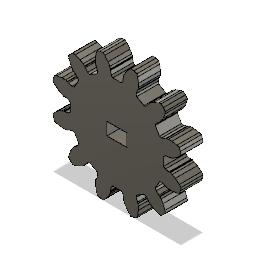
Motor Gear (Autodesk Fusion 360 design; units mm, degrees)
Autodesk Fusion 360 part; units mm, degrees
(part 1 of 2)
sketch "Sketch1" plane through (0, 0, 0) normal (0, 0, 1) x (1, 0, 0)
  circle A0 centre (141.6354, 183.0412) radius 17.7716
  line L0 (144.3354, 181.3412) -> (138.9354, 181.3412)
  line L1 (138.9354, 181.3412) -> (138.9354, 184.7412)
  line L2 (138.9354, 184.7412) -> (144.3354, 184.7412)
  line L3 (144.3354, 184.7412) -> (144.3354, 181.3412)
  line L4 (144.3354, 181.3412) -> (138.9354, 184.7412) construction
  line L5 (138.9354, 181.3412) -> (144.3354, 184.7412) construction
  line L6 (110, 165) -> (115.5, 165)
  line L7 (115.5, 165) -> (115.5, 168.5)
  line L8 (115.5, 168.5) -> (110, 168.5)
  line L9 (110, 168.5) -> (110, 165)
  line L10 (107, 171) -> (118, 171)
  line L11 (118, 171) -> (118, 162)
  line L12 (118, 162) -> (107, 162)
  line L13 (107, 162) -> (107, 171)
  arc A1 (143.6355, 181.3412) -> (143.8567, 181.6426) centre (141.6354, 183.0412) ccw
  arc A2 (143.8567, 184.4399) -> (143.6355, 184.7412) centre (141.6354, 183.0412) ccw
  arc A3 (139.6352, 184.7412) -> (139.414, 184.4399) centre (141.6354, 183.0412) ccw
  arc A4 (139.414, 181.6426) -> (139.6352, 181.3412) centre (141.6354, 183.0412) ccw
  point P0 (145.415, 200.4062)
  point P1 (137.8557, 165.6762)
  point P2 (141.6354, 183.0412)
  dimension "d1" = 5.25
  dimension "d6" = 5.4
  dimension "d7" = 3.4
  dimension "d8" = 5.5
  dimension "d9" = 3.5
  constraint coincident A0 P1
  constraint coincident A0 P0
  constraint concentric A0 A1
  constraint perpendicular L0 L1
  constraint parallel L0 L2
  constraint parallel L1 L3
  constraint horizontal L0
  constraint coincident L4 P2
  constraint coincident L5 P2
  constraint coincident P2 A0.centre
  constraint horizontal L6
  constraint vertical L7
  constraint horizontal L8
  constraint vertical L9
  constraint horizontal L10
  constraint vertical L11
  constraint horizontal L12
  constraint vertical L13
  constraint coincident L0 A4.end
  constraint coincident L0 A1.start
  constraint coincident L2 A2.end
  constraint coincident L2 A3.start
  constraint concentric A1 A3
  constraint coincident L4 A1.end
  constraint coincident L5 A2.start
  constraint concentric A1 A2
  constraint coincident L4 A3.end
  constraint coincident L5 A4.start
  constraint concentric A3 A4
  measures "d1" diameter of A1
  measures "d6" distance of L1.end L2.end
  measures "d7" distance of L0.end L1.end
  measures "d8" distance of L6.start L6.end
  measures "d9" distance of L6.start L8.end
sketch "30_12_Gears" plane through (0, 0, 0) normal (0, 0, 1) x (1, 0, 0)
  line L0 (152.0494, 175.714) -> (153.1879, 177.6861)
  line L1 (146.2489, 165.8233) -> (147.0446, 166.1129)
  line L2 (154.7859, 181.4961) -> (154.3178, 181.9027)
  line L3 (154.7841, 171.0855) -> (154.6561, 171.7367)
  line L4 (153.297, 174.2848) -> (153.2284, 174.3402)
  line L5 (154.2398, 170.4368) -> (154.7841, 171.0855)
  line L6 (150.2112, 171.6754) -> (150.3365, 171.4483)
  line L7 (142.7739, 170.3589) -> (143.1805, 169.8908)
  line L8 (154.9672, 177.352) -> (155.0495, 177.3202)
  line L9 (146.8725, 170.88) -> (146.9906, 171.4887)
  line L10 (156.5401, 177.1992) -> (157.9358, 177.4173)
  line L11 (156.1128, 181.2888) -> (156.0257, 181.3023)
  line L12 (158.8534, 178.4278) -> (159.0004, 179.2617)
  line L13 (153.0013, 174.4654) -> (152.2515, 175.1279)
  line L14 (152.2515, 175.1279) -> (152.0494, 175.714)
  line L15 (156.0257, 181.3023) -> (155.7665, 181.2973)
  line L16 (147.3246, 169.7094) -> (147.1906, 169.9314)
  line L17 (144.0283, 167.2123) -> (144.9151, 166.1127)
  line L18 (145.415, 165.6762) -> (146.2489, 165.8233)
  line L19 (147.4775, 168.1365) -> (147.4585, 169.1075)
  line L20 (151.6222, 170.5295) -> (152.94, 170.0205)
  line L21 (143.3743, 168.6509) -> (143.3879, 168.5638)
  line L22 (140.0902, 169.8908) -> (140.4968, 170.3589)
  line L23 (140.4968, 170.3589) -> (142.7739, 170.3589)
  line L24 (153.5912, 169.8926) -> (154.2398, 170.4368)
  line L25 (154.1472, 173.0544) -> (153.6453, 173.8858)
  line L26 (158.5637, 177.6321) -> (158.8534, 178.4278)
  line L27 (158.564, 179.7616) -> (157.4643, 180.6484)
  line L28 (154.6561, 171.7367) -> (154.1472, 173.0544)
  line L29 (153.2284, 174.3402) -> (153.0013, 174.4654)
  line L30 (155.0495, 177.3202) -> (155.5692, 177.2181)
  line L31 (147.2594, 166.7408) -> (147.4775, 168.1365)
  line L32 (148.9626, 172.6273) -> (149.5488, 172.4252)
  line L33 (147.3564, 169.6272) -> (147.3246, 169.7094)
  line L34 (147.4585, 169.1075) -> (147.3564, 169.6272)
  line L35 (156.614, 181.1174) -> (156.1128, 181.2888)
  line L36 (143.3793, 168.9102) -> (143.3743, 168.6509)
  line L37 (153.7966, 177.8041) -> (154.7452, 177.486)
  line L38 (143.1805, 169.8908) -> (143.3793, 168.9102)
  line L39 (144.9151, 166.1127) -> (145.415, 165.6762)
  line L40 (154.7452, 177.486) -> (154.9672, 177.352)
  line L41 (159.0004, 179.2617) -> (158.564, 179.7616)
  line L42 (155.5692, 177.2181) -> (156.5401, 177.1992)
  line L43 (153.6453, 173.8858) -> (153.297, 174.2848)
  line L44 (149.5488, 172.4252) -> (150.2112, 171.6754)
  line L45 (143.5593, 168.0627) -> (144.0283, 167.2123)
  line L46 (153.1879, 177.6861) -> (153.7966, 177.8041)
  line L47 (155.7665, 181.2973) -> (154.7859, 181.4961)
  line L48 (154.3178, 181.9027) -> (154.3178, 184.1798)
  line L49 (157.9358, 177.4173) -> (158.5637, 177.6321)
  line L50 (154.3178, 184.1798) -> (154.7859, 184.5864)
  line L51 (154.7859, 184.5864) -> (155.7665, 184.7852)
  line L52 (155.7665, 184.7852) -> (156.0257, 184.7801)
  line L53 (156.0257, 184.7801) -> (156.1128, 184.7937)
  line L54 (156.1128, 184.7937) -> (156.614, 184.9651)
  line L55 (140.4968, 195.7236) -> (140.0902, 196.1917)
  line L56 (145.415, 200.4062) -> (144.9151, 199.9698)
  line L57 (144.0283, 198.8702) -> (143.5593, 198.0198)
  line L58 (139.8829, 197.5187) -> (139.7115, 198.0198)
  line L59 (147.3246, 196.3731) -> (147.3564, 196.4553)
  line L60 (139.8914, 197.1723) -> (139.8965, 197.4316)
  line L61 (155.0495, 188.7622) -> (154.9672, 188.7305)
  line L62 (151.6222, 195.553) -> (150.7908, 195.0511)
  line L63 (152.2515, 190.9546) -> (153.0013, 191.6171)
  line L64 (150.3365, 194.6342) -> (150.2112, 194.4071)
  line L65 (154.9672, 188.7305) -> (154.7452, 188.5965)
  line L66 (153.0013, 191.6171) -> (153.2284, 191.7423)
  line L67 (157.4643, 180.6484) -> (156.614, 181.1174)
  line L68 (150.3918, 194.7028) -> (150.3365, 194.6342)
  line L69 (153.6453, 192.1967) -> (154.1472, 193.0281)
  line L70 (159.0004, 186.8208) -> (158.8534, 187.6547)
  line L71 (150.7908, 195.0511) -> (150.3918, 194.7028)
  line L72 (153.7966, 188.2783) -> (153.1879, 188.3964)
  line L73 (154.2398, 195.6457) -> (153.5912, 196.1899)
  line L74 (152.94, 196.062) -> (151.6222, 195.553)
  line L75 (147.1906, 196.1511) -> (147.3246, 196.3731)
  line L76 (148.9626, 193.4552) -> (146.9906, 194.5938)
  line L77 (153.2284, 191.7423) -> (153.297, 191.7977)
  line L78 (153.297, 191.7977) -> (153.6453, 192.1967)
  line L79 (153.5912, 196.1899) -> (152.94, 196.062)
  line L80 (143.5593, 198.0198) -> (143.3879, 197.5187)
  line L81 (158.5637, 188.4504) -> (157.9358, 188.6652)
  line L82 (155.5692, 188.8644) -> (155.0495, 188.7622)
  line L83 (156.614, 184.9651) -> (157.4643, 185.4341)
  line L84 (149.5488, 193.6573) -> (148.9626, 193.4552)
  line L85 (146.9906, 194.5938) -> (146.8725, 195.2025)
  line L86 (156.5401, 188.8833) -> (155.5692, 188.8644)
  line L87 (154.7452, 188.5965) -> (153.7966, 188.2783)
  line L88 (140.0902, 196.1917) -> (139.8914, 197.1723)
  line L89 (158.8534, 187.6547) -> (158.5637, 188.4504)
  line L90 (154.1472, 193.0281) -> (154.6561, 194.3458)
  line L91 (154.6561, 194.3458) -> (154.7841, 194.997)
  line L92 (150.2112, 194.4071) -> (149.5488, 193.6573)
  line L93 (152.0494, 190.3685) -> (152.2515, 190.9546)
  line L94 (154.7841, 194.997) -> (154.2398, 195.6457)
  line L95 (157.9358, 188.6652) -> (156.5401, 188.8833)
  line L96 (153.1879, 188.3964) -> (152.0494, 190.3685)
  line L97 (157.4643, 185.4341) -> (158.564, 186.3209)
  line L98 (158.564, 186.3209) -> (159.0004, 186.8208)
  line L99 (146.8725, 195.2025) -> (147.1906, 196.1511)
  line L100 (147.3564, 196.4553) -> (147.4585, 196.975)
  line L101 (142.7739, 195.7236) -> (140.4968, 195.7236)
  line L102 (147.4775, 197.946) -> (147.2594, 199.3417)
  line L103 (129.9738, 191.7977) -> (130.0424, 191.7423)
  line L104 (130.3307, 196.062) -> (129.6796, 196.1899)
  line L105 (133.0595, 194.4071) -> (132.9342, 194.6342)
  line L106 (133.722, 193.6573) -> (133.0595, 194.4071)
  line L107 (124.707, 188.4504) -> (124.707, 188.4504)
  line L108 (130.2695, 191.6171) -> (131.0193, 190.9546)
  line L109 (127.7016, 188.8644) -> (126.7306, 188.8833)
  line L110 (124.707, 188.4504) -> (124.707, 188.4504)
  line L111 (131.0193, 190.9546) -> (131.2214, 190.3685)
  line L112 (136.2802, 194.5938) -> (134.3081, 193.4552)
  line L113 (128.4866, 194.997) -> (128.6146, 194.3458)
  line L114 (131.2214, 190.3685) -> (130.0828, 188.3964)
  line L115 (131.6485, 195.553) -> (130.3307, 196.062)
  line L116 (143.3743, 197.4316) -> (143.3793, 197.1723)
  line L117 (134.3081, 193.4552) -> (133.722, 193.6573)
  line L118 (139.7115, 198.0198) -> (139.2424, 198.8702)
  line L119 (144.9151, 199.9698) -> (144.0283, 198.8702)
  line L120 (146.2489, 200.2592) -> (145.415, 200.4062)
  line L121 (132.9342, 194.6342) -> (132.8789, 194.7028)
  line L122 (136.0114, 199.3417) -> (135.7933, 197.946)
  line L123 (139.8965, 197.4316) -> (139.8829, 197.5187)
  line L124 (132.8789, 194.7028) -> (132.4799, 195.0511)
  line L125 (129.4741, 188.2783) -> (128.5255, 188.5965)
  line L126 (130.0828, 188.3964) -> (129.4741, 188.2783)
  line L127 (147.4585, 196.975) -> (147.4775, 197.946)
  line L128 (128.6146, 194.3458) -> (129.1236, 193.0281)
  line L129 (130.0424, 191.7423) -> (130.2695, 191.6171)
  line L130 (138.3557, 199.9698) -> (137.8557, 200.4062)
  line L131 (135.9461, 196.3731) -> (136.0801, 196.1511)
  line L132 (139.2424, 198.8702) -> (138.3557, 199.9698)
  line L133 (143.3793, 197.1723) -> (143.1805, 196.1917)
  line L134 (137.8557, 200.4062) -> (137.0218, 200.2592)
  line L135 (143.3879, 197.5187) -> (143.3743, 197.4316)
  line L136 (136.2261, 199.9696) -> (136.0114, 199.3417)
  line L137 (135.7933, 197.946) -> (135.8122, 196.975)
  line L138 (129.6796, 196.1899) -> (129.0309, 195.6457)
  line L139 (147.0446, 199.9696) -> (146.2489, 200.2592)
  line L140 (143.1805, 196.1917) -> (142.7739, 195.7236)
  line L141 (147.2594, 199.3417) -> (147.0446, 199.9696)
  line L142 (137.0218, 200.2592) -> (136.2261, 199.9696)
  line L143 (129.1236, 193.0281) -> (129.6255, 192.1967)
  line L144 (128.5255, 188.5965) -> (128.3035, 188.7305)
  line L145 (135.8122, 196.975) -> (135.9143, 196.4553)
  line L146 (136.0801, 196.1511) -> (136.3982, 195.2025)
  line L147 (129.0309, 195.6457) -> (128.4866, 194.997)
  line L148 (132.4799, 195.0511) -> (131.6485, 195.553)
  line L149 (128.3035, 188.7305) -> (128.2213, 188.7622)
  line L150 (135.9143, 196.4553) -> (135.9461, 196.3731)
  line L151 (129.6255, 192.1967) -> (129.9738, 191.7977)
  line L152 (136.3982, 195.2025) -> (136.2802, 194.5938)
  line L153 (128.2213, 188.7622) -> (127.7016, 188.8644)
  line L154 (126.7306, 188.8833) -> (125.3349, 188.6652)
  line L155 (124.5194, 177.6472) -> (123.9642, 177.8157)
  line L156 (123.8799, 180.6066) -> (124.2682, 180.7082)
  line L157 (125.0362, 177.45) -> (124.5194, 177.6472)
  line L158 (126.4909, 176.7057) -> (125.6979, 177.1431)
  line L159 (123.6055, 177.9958) -> (123.446, 178.1876)
  line L160 (124.2682, 180.7082) -> (124.8463, 180.7576)
  line L161 (125.6979, 177.1431) -> (125.0362, 177.45)
  line L162 (125.3928, 180.843) -> (126.1039, 181.0056)
  line L163 (127.7577, 173.6189) -> (128.0126, 174.5701)
  line L164 (128.0126, 174.5701) -> (128.1667, 175.5427)
  line L165 (127.3994, 176.1183) -> (126.4909, 176.7057)
  line L166 (125.3349, 188.6652) -> (124.707, 188.4504)
  line L167 (124.8463, 180.7576) -> (125.3928, 180.843)
  line L168 (123.9642, 177.8157) -> (123.6055, 177.9958)
  line L169 (128.1667, 175.5427) -> (127.3994, 176.1183)
  line L170 (123.446, 178.1876) -> (123.684, 180.4522)
  line L171 (123.684, 180.4522) -> (123.8799, 180.6066)
  line L172 (123.5698, 192.9026) -> (122.9941, 192.8307)
  line L173 (125.0362, 188.6323) -> (125.6979, 188.9392)
  line L174 (128.8514, 182.0578) -> (128.903, 183.0412)
  line L175 (122.5932, 192.8493) -> (122.3694, 192.9596)
  line L176 (124.2682, 185.3741) -> (123.8799, 185.4758)
  line L177 (128.1667, 190.5397) -> (128.0126, 191.5122)
  line L178 (127.9813, 181.6542) -> (128.8514, 182.0578)
  line L179 (127.9813, 184.4281) -> (126.9705, 184.8137)
  line L180 (123.8799, 185.4758) -> (123.684, 185.6301)
  line L181 (126.9705, 181.2686) -> (127.9813, 181.6542)
  line L182 (126.1039, 181.0056) -> (126.9705, 181.2686)
  line L183 (125.7538, 192.8443) -> (124.8515, 192.9214)
  line L184 (128.903, 183.0412) -> (128.8514, 184.0246)
  line L185 (126.9705, 184.8137) -> (126.1039, 185.0767)
  line L186 (126.1039, 185.0767) -> (125.3928, 185.2393)
  line L187 (124.5194, 188.4352) -> (125.0362, 188.6323)
  line L188 (123.446, 187.8948) -> (123.6055, 188.0865)
  line L189 (124.8515, 192.9214) -> (124.1222, 192.9327)
  line L190 (125.6979, 188.9392) -> (126.4909, 189.3766)
  line L191 (123.9642, 188.2667) -> (124.5194, 188.4352)
  line L192 (126.4909, 189.3766) -> (127.3994, 189.964)
  line L193 (124.1222, 192.9327) -> (123.5698, 192.9026)
  line L194 (126.8227, 192.6773) -> (125.7538, 192.8443)
  line L195 (125.3928, 185.2393) -> (124.8463, 185.3247)
  line L196 (122.9941, 192.8307) -> (122.5932, 192.8493)
  line L197 (124.8463, 185.3247) -> (124.2682, 185.3741)
  line L198 (123.6055, 188.0865) -> (123.9642, 188.2667)
  line L199 (128.0126, 191.5122) -> (127.7577, 192.4634)
  line L200 (122.3694, 192.9596) -> (121.6657, 195.1252)
  line L201 (114.0546, 208.3143) -> (114.4047, 208.7769)
  line L202 (115.4463, 210.6974) -> (115.8361, 211.7066)
  line L203 (116.4975, 206.4527) -> (116.0007, 206.1528)
  line L204 (112.0365, 212.6016) -> (111.4399, 212.182)
  line L205 (110.2518, 211.2158) -> (110.006, 211.1735)
  line L206 (110.006, 211.1735) -> (108.1637, 212.512)
  line L207 (110.5871, 211.4364) -> (110.2518, 211.2158)
  line L208 (115.3776, 206.0166) -> (113.8539, 207.7088)
  line L209 (119.182, 202.7578) -> (119.5739, 203.1482)
  line L210 (118.4889, 202.0676) -> (118.7433, 202.3781)
  line L211 (113.8703, 207.9577) -> (114.0546, 208.3143)
  line L212 (124.9334, 200.4905) -> (123.9744, 200.5053)
  line L213 (113.8539, 207.7088) -> (113.8703, 207.9577)
  line L214 (108.128, 212.7588) -> (108.2341, 213.1459)
  line L215 (116.0007, 206.1528) -> (115.6269, 206.0068)
  line L216 (118.7433, 202.3781) -> (119.182, 202.7578)
  line L217 (120.6001, 204.4198) -> (121.1912, 205.3259)
  line L218 (122.0953, 195.5967) -> (122.6034, 195.877)
  line L219 (123.9744, 200.5053) -> (122.8941, 200.4464)
  line L220 (121.1912, 205.3259) -> (121.6579, 206.1638)
  line L221 (120.1975, 199.8592) -> (119.8015, 199.7942)
  line L222 (121.1216, 206.9897) -> (120.5019, 207.755)
  line L223 (119.5597, 199.8555) -> (118.4211, 201.8275)
  line L224 (111.0107, 211.8329) -> (110.5871, 211.4364)
  line L225 (120.0536, 203.6977) -> (120.6001, 204.4198)
  line L226 (122.8941, 200.4464) -> (121.9955, 200.3342)
  line L227 (118.5163, 207.2878) -> (117.6607, 206.9912)
  line L228 (121.7819, 195.346) -> (122.0953, 195.5967)
  line L229 (123.0679, 196.1773) -> (123.6513, 196.6151)
  line L230 (118.4211, 201.8275) -> (118.4889, 202.0676)
  line L231 (121.9955, 200.3342) -> (121.2798, 200.1935)
  line L232 (121.2798, 200.1935) -> (120.7457, 200.0493)
  line L233 (123.684, 185.6301) -> (123.446, 187.8948)
  line L234 (124.336, 197.2078) -> (125.1026, 197.9712)
  line L235 (125.3805, 199.6131) -> (124.9334, 200.4905)
  line L236 (121.6657, 195.1252) -> (121.7819, 195.346)
  line L237 (125.1026, 197.9712) -> (125.7334, 198.6938)
  line L238 (119.5739, 203.1482) -> (120.0536, 203.6977)
  line L239 (120.7457, 200.0493) -> (120.1975, 199.8592)
  line L240 (121.6579, 206.1638) -> (121.1216, 206.9897)
  line L241 (120.5019, 207.755) -> (119.5607, 207.57)
  line L242 (119.8015, 199.7942) -> (119.5597, 199.8555)
  line L243 (125.7334, 198.6938) -> (125.3805, 199.6131)
  line L244 (127.3994, 189.964) -> (128.1667, 190.5397)
  line L245 (115.0619, 209.8775) -> (115.4463, 210.6974)
  line L246 (127.7577, 192.4634) -> (126.8227, 192.6773)
  line L247 (128.8514, 184.0246) -> (127.9813, 184.4281)
  line L248 (122.6034, 195.877) -> (123.0679, 196.1773)
  line L249 (119.5607, 207.57) -> (118.5163, 207.2878)
  line L250 (123.6513, 196.6151) -> (124.336, 197.2078)
  line L251 (94.15, 220.5651) -> (93.979, 221.4545)
  line L252 (96.8821, 217.7658) -> (96.6748, 217.6272)
  line L253 (101.5993, 216.0271) -> (101.513, 216.2612)
  line L254 (108.8944, 214.8844) -> (109.1, 215.7664)
  line L255 (85.8653, 221.825) -> (85.3761, 222.79)
  line L256 (94.2374, 219.841) -> (94.15, 220.5651)
  line L257 (93.979, 221.4545) -> (93.7012, 222.5)
  line L258 (115.4221, 213.3196) -> (114.6568, 213.9393)
  line L259 (99.7986, 222.0456) -> (99.1459, 221.3427)
  line L260 (108.5311, 218.3262) -> (107.6537, 218.7733)
  line L261 (101.513, 216.2612) -> (101.5363, 216.6619)
  line L262 (82.3396, 221.4545) -> (82.1686, 220.5651)
  line L263 (104.1934, 215.4789) -> (103.9112, 215.1934)
  line L264 (109.357, 217.7899) -> (108.5311, 218.3262)
  line L265 (111.4399, 212.182) -> (111.0107, 211.8329)
  line L266 (113.7747, 213.5627) -> (112.8118, 213.0696)
  line L267 (104.8724, 216.3855) -> (104.5252, 215.9548)
  line L268 (93.7012, 222.5) -> (93.3908, 223.4076)
  line L269 (107.6537, 218.7733) -> (106.8692, 218.2215)
  line L270 (108.6797, 214.1873) -> (108.8944, 214.8844)
  line L271 (112.8118, 213.0696) -> (112.0365, 212.6016)
  line L272 (109.2714, 216.8345) -> (109.357, 217.7899)
  line L273 (105.3688, 216.9199) -> (104.8724, 216.3855)
  line L274 (101.6691, 221.4378) -> (100.7498, 221.7907)
  line L275 (101.8384, 219.4051) -> (101.784, 220.4855)
  line L276 (101.5363, 216.6619) -> (101.668, 217.2269)
  line L277 (116.9898, 206.7049) -> (116.4975, 206.4527)
  line L278 (96.6748, 217.6272) -> (94.4474, 218.1006)
  line L279 (115.8361, 211.7066) -> (116.1184, 212.6233)
  line L280 (106.8692, 218.2215) -> (106.0298, 217.5389)
  line L281 (101.784, 220.4855) -> (101.6691, 221.4378)
  line L282 (94.4474, 218.1006) -> (94.3144, 218.3116)
  line L283 (114.6569, 213.9393) -> (113.7747, 213.5627)
  line L284 (108.4804, 213.6713) -> (108.6797, 214.1873)
  line L285 (97.0988, 218.1037) -> (96.8821, 217.7658)
  line L286 (101.7557, 217.7731) -> (101.8207, 218.4996)
  line L287 (89.7231, 219.7659) -> (89.6135, 219.1961)
  line L288 (98.4668, 220.5006) -> (97.9489, 219.7577)
  line L289 (90.4533, 221.825) -> (90.1012, 220.9907)
  line L290 (106.0298, 217.5389) -> (105.3688, 216.9199)
  line L291 (90.1012, 220.9907) -> (89.8651, 220.3005)
  line L292 (94.2539, 218.7084) -> (94.2652, 219.2885)
  line L293 (90.9425, 222.79) -> (90.4533, 221.825)
  line L294 (101.668, 217.2269) -> (101.7557, 217.7731)
  line L295 (117.6607, 206.9912) -> (116.9898, 206.7049)
  line L296 (97.9489, 219.7577) -> (97.5745, 219.1317)
  line L297 (97.3244, 218.6383) -> (97.0988, 218.1037)
  line L298 (104.5252, 215.9548) -> (104.1934, 215.4789)
  line L299 (92.4182, 223.5616) -> (91.4348, 223.6132)
  line L300 (103.6795, 215.1009) -> (101.5993, 216.0271)
  line L301 (87.0207, 218.6419) -> (86.8467, 218.8206)
  line L302 (108.2341, 213.1459) -> (108.4804, 213.6713)
  line L303 (116.1184, 212.6233) -> (115.4221, 213.3196)
  line L304 (108.1637, 212.512) -> (108.128, 212.7588)
  line L305 (115.6269, 206.0068) -> (115.3776, 206.0166)
  line L306 (99.1459, 221.3427) -> (98.4668, 220.5006)
  line L307 (101.8207, 218.4996) -> (101.8384, 219.4051)
  line L308 (114.707, 209.2402) -> (115.0619, 209.8775)
  line L309 (114.4047, 208.7769) -> (114.707, 209.2402)
  line L310 (109.1, 215.7664) -> (109.2714, 216.8345)
  line L311 (97.5745, 219.1317) -> (97.3244, 218.6383)
  line L312 (100.7498, 221.7907) -> (99.7986, 222.0456)
  line L313 (103.9112, 215.1934) -> (103.6795, 215.1009)
  line L314 (85.3761, 222.79) -> (84.8838, 223.6132)
  line L315 (74.5629, 148.3094) -> (74.4978, 147.5829)
  line L316 (94.4474, 147.9819) -> (96.6748, 148.4554)
  line L317 (82.0647, 147.3741) -> (82.0534, 146.794)
  line L318 (93.3908, 142.675) -> (93.7012, 143.5825)
  line L319 (75.5688, 144.2918) -> (76.52, 144.037)
  line L320 (86.2174, 145.0919) -> (86.4534, 145.782)
  line L321 (82.0534, 146.794) -> (82.0812, 146.2415)
  line L322 (82.9278, 142.675) -> (83.9004, 142.5209)
  line L323 (82.3396, 144.6281) -> (82.6174, 143.5825)
  line L324 (78.7441, 146.9509) -> (78.9942, 147.4443)
  line L325 (81.8712, 147.9819) -> (82.0042, 147.7709)
  line L326 (74.6495, 144.6447) -> (75.5688, 144.2918)
  line L327 (78.9942, 147.4443) -> (79.2198, 147.9788)
  line L328 (74.5346, 145.597) -> (74.6495, 144.6447)
  line L329 (74.4802, 146.6775) -> (74.5346, 145.597)
  line L330 (74.6506, 148.8556) -> (74.5629, 148.3094)
  line L331 (82.6174, 143.5825) -> (82.9278, 142.675)
  line L332 (82.0042, 147.7709) -> (82.0647, 147.3741)
  line L333 (85.8653, 144.2575) -> (86.2174, 145.0919)
  line L334 (83.9004, 142.5209) -> (84.8838, 142.4694)
  line L335 (85.3761, 143.2926) -> (85.8653, 144.2575)
  line L336 (76.52, 144.037) -> (77.1727, 144.7398)
  line L337 (78.3697, 146.3249) -> (78.7441, 146.9509)
  line L338 (74.4978, 147.5829) -> (74.4802, 146.6775)
  line L339 (77.1727, 144.7398) -> (77.8518, 145.582)
  line L340 (86.4534, 145.782) -> (86.5955, 146.3166)
  line L341 (86.5955, 146.3166) -> (86.705, 146.8864)
  line L342 (91.4348, 142.4694) -> (92.4182, 142.5209)
  line L343 (82.1686, 145.5174) -> (82.3396, 144.6281)
  line L344 (82.0812, 146.2415) -> (82.1686, 145.5174)
  line L345 (79.2198, 147.9788) -> (79.4364, 148.3167)
  line L346 (93.979, 144.6281) -> (94.15, 145.5174)
  line L347 (77.8518, 145.582) -> (78.3697, 146.3249)
  line L348 (79.6438, 148.4554) -> (81.8712, 147.9819)
  line L349 (84.8838, 142.4694) -> (85.3761, 143.2926)
  line L350 (79.4364, 148.3167) -> (79.6438, 148.4554)
  line L351 (89.7231, 146.3166) -> (89.8651, 145.782)
  line L352 (86.8467, 147.2619) -> (87.0207, 147.4407)
  line L353 (94.15, 145.5174) -> (94.2374, 146.2415)
  line L354 (103.6795, 150.9816) -> (103.9112, 150.8891)
  line L355 (107.6537, 147.3093) -> (108.5311, 147.7563)
  line L356 (97.5745, 146.9509) -> (97.9489, 146.3249)
  line L357 (108.5311, 147.7563) -> (109.357, 148.2926)
  line L358 (101.6691, 144.6447) -> (101.784, 145.597)
  line L359 (97.0988, 147.9788) -> (97.3244, 147.4443)
  line L360 (86.705, 146.8864) -> (86.8467, 147.2619)
  line L361 (94.2652, 146.794) -> (94.2539, 147.3741)
  line L362 (89.4719, 147.2619) -> (89.6135, 146.8864)
  line L363 (96.6748, 148.4554) -> (96.8821, 148.3167)
  line L364 (97.9489, 146.3249) -> (98.4668, 145.582)
  line L365 (109.2714, 149.248) -> (109.1, 150.3162)
  line L366 (99.7986, 144.037) -> (100.7498, 144.2918)
  line L367 (104.5252, 150.1277) -> (104.8724, 149.6971)
  line L368 (94.2374, 146.2415) -> (94.2652, 146.794)
  line L369 (109.1, 150.3162) -> (108.8944, 151.1982)
  line L370 (101.513, 149.8214) -> (101.5993, 150.0554)
  line L371 (108.4804, 152.4113) -> (108.2341, 152.9366)
  line L372 (104.1934, 150.6037) -> (104.5252, 150.1277)
  line L373 (89.6135, 146.8864) -> (89.7231, 146.3166)
  line L374 (94.3144, 147.7709) -> (94.4474, 147.9819)
  line L375 (97.3244, 147.4443) -> (97.5745, 146.9509)
  line L376 (90.9425, 143.2926) -> (91.4348, 142.4694)
  line L377 (99.1459, 144.7398) -> (99.7986, 144.037)
  line L378 (98.4668, 145.582) -> (99.1459, 144.7398)
  line L379 (108.2341, 152.9366) -> (108.128, 153.3237)
  line L380 (89.8651, 145.782) -> (90.1012, 145.0919)
  line L381 (89.2978, 147.4407) -> (89.4719, 147.2619)
  line L382 (108.1637, 153.5706) -> (110.006, 154.909)
  line L383 (90.1012, 145.0919) -> (90.4533, 144.2575)
  line L384 (96.8821, 148.3167) -> (97.0988, 147.9788)
  line L385 (101.8207, 147.5829) -> (101.7557, 148.3094)
  line L386 (106.0298, 148.5436) -> (106.8692, 147.861)
  line L387 (106.8692, 147.861) -> (107.6537, 147.3093)
  line L388 (100.7498, 144.2918) -> (101.6691, 144.6447)
  line L389 (90.4533, 144.2575) -> (90.9425, 143.2926)
  line L390 (87.0207, 147.4407) -> (89.2978, 147.4407)
  line L391 (92.4182, 142.5209) -> (93.3908, 142.675)
  line L392 (93.7012, 143.5825) -> (93.979, 144.6281)
  line L393 (94.2539, 147.3741) -> (94.3144, 147.7709)
  line L394 (108.6797, 151.8952) -> (108.4804, 152.4113)
  line L395 (113.8539, 158.3737) -> (115.3776, 160.066)
  line L396 (115.4463, 155.3851) -> (115.0619, 156.2051)
  line L397 (101.5363, 149.4207) -> (101.513, 149.8214)
  line L398 (111.4399, 153.9006) -> (112.0365, 153.481)
  line L399 (116.0007, 159.9295) -> (116.4975, 159.6297)
  line L400 (119.182, 163.3246) -> (118.7433, 163.7044)
  line L401 (116.9898, 159.3775) -> (117.6607, 159.0911)
  line L402 (110.006, 154.909) -> (110.2518, 154.8667)
  line L403 (104.8724, 149.6971) -> (105.3688, 149.1626)
  line L404 (115.6269, 160.0756) -> (116.0007, 159.9295)
  line L405 (114.0546, 157.7683) -> (113.8703, 158.1248)
  line L406 (101.5993, 150.0554) -> (103.6795, 150.9816)
  line L407 (108.128, 153.3237) -> (108.1637, 153.5706)
  line L408 (101.784, 145.597) -> (101.8384, 146.6775)
  line L409 (103.9112, 150.8891) -> (104.1934, 150.6037)
  line L410 (105.3688, 149.1626) -> (106.0298, 148.5436)
  line L411 (111.0107, 154.2496) -> (111.4399, 153.9006)
  line L412 (119.5607, 158.5124) -> (120.5019, 158.3274)
  line L413 (115.0619, 156.2051) -> (114.707, 156.8423)
  line L414 (113.7747, 152.5198) -> (114.6569, 152.1432)
  line L415 (116.4975, 159.6297) -> (116.9898, 159.3775)
  line L416 (101.7557, 148.3094) -> (101.668, 148.8556)
  line L417 (110.5871, 154.6462) -> (111.0107, 154.2496)
  line L418 (101.668, 148.8556) -> (101.5363, 149.4207)
  line L419 (108.8944, 151.1982) -> (108.6797, 151.8952)
  line L420 (121.1216, 159.0927) -> (121.6579, 159.9186)
  line L421 (101.8384, 146.6775) -> (101.8207, 147.5829)
  line L422 (116.1184, 153.4592) -> (115.8361, 154.3759)
  line L423 (112.0365, 153.481) -> (112.8118, 153.013)
  line L424 (109.357, 148.2926) -> (109.2714, 149.248)
  line L425 (110.2518, 154.8667) -> (110.5871, 154.6462)
  line L426 (121.1912, 160.7565) -> (120.6001, 161.6626)
  line L427 (112.8118, 153.013) -> (113.7747, 152.5198)
  line L428 (114.4047, 157.3056) -> (114.0546, 157.7683)
  line L429 (123.0679, 169.905) -> (122.6034, 170.2053)
  line L430 (119.5739, 162.9343) -> (119.182, 163.3246)
  line L431 (125.7334, 167.3885) -> (125.1026, 168.1111)
  line L432 (123.5698, 173.1798) -> (124.1222, 173.1497)
  line L433 (123.6513, 169.4672) -> (123.0679, 169.905)
  line L434 (118.5163, 158.7946) -> (119.5607, 158.5124)
  line L435 (118.4889, 164.0148) -> (118.4211, 164.2549)
  line L436 (124.1222, 173.1497) -> (124.8515, 173.161)
  line L437 (126.8227, 173.4051) -> (127.7577, 173.6189)
  line L438 (117.6607, 159.0911) -> (118.5163, 158.7946)
  line L439 (86.2572, 182.4231) -> (86.1702, 182.8321)
  line L440 (90.0614, 182.4231) -> (89.8913, 182.0412)
  line L441 (89.3349, 184.6592) -> (89.6456, 184.3794)
  line L442 (120.1975, 166.2232) -> (120.7457, 166.0331)
  line L443 (115.4221, 152.7629) -> (116.1184, 153.4592)
  line L444 (114.707, 156.8423) -> (114.4047, 157.3056)
  line L445 (113.8703, 158.1248) -> (113.8539, 158.3737)
  line L446 (120.0536, 162.3847) -> (119.5739, 162.9343)
  line L447 (115.8361, 154.3759) -> (115.4463, 155.3851)
  line L448 (122.3694, 173.1228) -> (122.5932, 173.233)
  line L449 (124.336, 168.8745) -> (123.6513, 169.4672)
  line L450 (125.1026, 168.1111) -> (124.336, 168.8745)
  line L451 (120.7457, 166.0331) -> (121.2798, 165.8889)
  line L452 (127.7577, 173.6189) -> (127.7577, 173.6189)
  line L453 (124.9334, 165.5918) -> (125.3805, 166.4692)
  line L454 (125.3805, 166.4692) -> (125.7334, 167.3885)
  line L455 (124.8515, 173.161) -> (125.7538, 173.238)
  line L456 (122.0953, 170.4856) -> (121.7819, 170.7364)
  line L457 (127.7577, 173.6189) -> (127.7577, 173.6189)
  line L458 (119.5597, 166.2269) -> (119.8015, 166.2882)
  line L459 (120.5019, 158.3274) -> (121.1216, 159.0927)
  line L460 (118.7433, 163.7044) -> (118.4889, 164.0148)
  line L461 (114.6569, 152.1432) -> (115.4221, 152.7629)
  line L462 (118.4211, 164.2549) -> (119.5597, 166.2269)
  line L463 (115.3776, 160.066) -> (115.6269, 160.0756)
  line L464 (121.6657, 170.9571) -> (122.3694, 173.1228)
  line L465 (122.6034, 170.2053) -> (122.0953, 170.4856)
  line L466 (123.9744, 165.5771) -> (124.9334, 165.5918)
  line L467 (122.9941, 173.2516) -> (123.5698, 173.1798)
  line L468 (121.7819, 170.7364) -> (121.6657, 170.9571)
  line L469 (122.8941, 165.636) -> (123.9744, 165.5771)
  line L470 (121.6579, 159.9186) -> (121.1912, 160.7565)
  line L471 (120.6001, 161.6626) -> (120.0536, 162.3847)
  line L472 (121.9955, 165.7482) -> (122.8941, 165.636)
  line L473 (122.5932, 173.233) -> (122.9941, 173.2516)
  line L474 (125.7538, 173.238) -> (126.8227, 173.4051)
  line L475 (121.2798, 165.8889) -> (121.9955, 165.7482)
  line L476 (119.8015, 166.2882) -> (120.1975, 166.2232)
  line L477 (88.5751, 181.0849) -> (88.1593, 181.0412)
  line L478 (88.9728, 181.2141) -> (88.5751, 181.0849)
  line L479 (89.6456, 181.7029) -> (89.3349, 181.4231)
  line L480 (130.0828, 177.6861) -> (131.2214, 175.714)
  line L481 (131.2214, 175.714) -> (131.0193, 175.1279)
  line L482 (124.7067, 179.7616) -> (124.2703, 179.2617)
  line L483 (127.5043, 181.2973) -> (127.245, 181.3023)
  line L484 (131.0193, 175.1279) -> (130.2695, 174.4654)
  line L485 (130.2695, 174.4654) -> (130.0424, 174.3402)
  line L486 (88.5751, 181.0849) -> (88.5751, 181.0849)
  line L487 (89.3349, 181.4231) -> (88.9728, 181.2141)
  line L488 (128.3035, 177.352) -> (128.5255, 177.486)
  line L489 (128.953, 181.9027) -> (128.4849, 181.4961)
  line L490 (89.8913, 184.0412) -> (90.0614, 183.6592)
  line L491 (88.1593, 185.0412) -> (88.5751, 184.9975)
  line L492 (86.1702, 183.2502) -> (86.2572, 183.6592)
  line L493 (90.1483, 182.8321) -> (90.0614, 182.4231)
  line L494 (86.1702, 182.8321) -> (86.1702, 183.2502)
  line L495 (128.4849, 184.5864) -> (128.953, 184.1798)
  line L496 (89.8913, 182.0412) -> (89.6456, 181.7029)
  line L497 (126.7306, 177.1992) -> (127.7016, 177.2181)
  line L498 (90.0614, 183.6592) -> (90.1483, 183.2502)
  line L499 (88.5751, 181.0849) -> (88.5751, 181.0849)
  line L500 (128.953, 184.1798) -> (128.953, 181.9027)
  line L501 (86.2572, 183.6592) -> (86.4272, 184.0412)
  line L502 (128.5255, 177.486) -> (129.4741, 177.8041)
  line L503 (86.4272, 184.0412) -> (86.673, 184.3794)
  line L504 (90.1483, 183.2502) -> (90.1483, 182.8321)
  line L505 (88.5751, 184.9975) -> (88.9728, 184.8683)
  line L506 (86.4272, 182.0412) -> (86.2572, 182.4231)
  line L507 (86.9837, 184.6592) -> (87.3458, 184.8683)
  line L508 (86.9837, 181.4231) -> (86.673, 181.7029)
  line L509 (124.2703, 186.8208) -> (124.7067, 186.3209)
  line L510 (124.707, 177.6321) -> (125.3349, 177.4173)
  line L511 (126.6568, 184.9651) -> (127.1579, 184.7937)
  line L512 (128.2213, 177.3202) -> (128.3035, 177.352)
  line L513 (86.673, 181.7029) -> (86.4272, 182.0412)
  line L514 (127.1579, 184.7937) -> (127.245, 184.7801)
  line L515 (125.3349, 177.4173) -> (126.7306, 177.1992)
  line L516 (88.1593, 181.0412) -> (87.7435, 181.0849)
  line L517 (89.6456, 184.3794) -> (89.8913, 184.0412)
  line L518 (87.7435, 184.9975) -> (88.1593, 185.0412)
  line L519 (86.673, 184.3794) -> (86.9837, 184.6592)
  line L520 (87.3458, 184.8683) -> (87.7435, 184.9975)
  line L521 (127.1579, 181.2888) -> (126.6568, 181.1174)
  line L522 (127.5043, 184.7852) -> (128.4849, 184.5864)
  line L523 (129.4741, 177.8041) -> (130.0828, 177.6861)
  line L524 (124.707, 188.4504) -> (124.4174, 187.6547)
  line L525 (87.3458, 181.2141) -> (86.9837, 181.4231)
  line L526 (88.9728, 184.8683) -> (89.3349, 184.6592)
  line L527 (87.7435, 181.0849) -> (87.3458, 181.2141)
  line L528 (127.245, 181.3023) -> (127.1579, 181.2888)
  line L529 (127.7016, 177.2181) -> (128.2213, 177.3202)
  line L530 (125.8064, 180.6484) -> (124.7067, 179.7616)
  line L531 (130.0424, 174.3402) -> (129.9738, 174.2848)
  line L532 (129.0309, 170.4368) -> (129.6796, 169.8926)
  line L533 (137.8557, 165.6762) -> (138.3557, 166.1127)
  line L534 (136.3982, 170.88) -> (136.0801, 169.9314)
  line L535 (134.3081, 172.6273) -> (136.2802, 171.4887)
  line L536 (135.8122, 169.1075) -> (135.7933, 168.1365)
  line L537 (129.1236, 173.0544) -> (128.6146, 171.7367)
  line L538 (150.3918, 171.3797) -> (150.7908, 171.0314)
  line L539 (136.0114, 166.7408) -> (136.2261, 166.1129)
  line L540 (136.2802, 171.4887) -> (136.3982, 170.88)
  line L541 (135.9461, 169.7094) -> (135.9143, 169.6272)
  line L542 (129.9738, 174.2848) -> (129.6255, 173.8858)
  line L543 (136.2261, 166.1129) -> (137.0218, 165.8233)
  line L544 (147.1906, 169.9314) -> (146.8725, 170.88)
  line L545 (128.4849, 181.4961) -> (127.5043, 181.2973)
  line L546 (127.245, 184.7801) -> (127.5043, 184.7852)
  line L547 (152.94, 170.0205) -> (153.5912, 169.8926)
  line L548 (137.0218, 165.8233) -> (137.8557, 165.6762)
  line L549 (150.3365, 171.4483) -> (150.3918, 171.3797)
  line L550 (138.3557, 166.1127) -> (139.2424, 167.2123)
  line L551 (128.4866, 171.0855) -> (129.0309, 170.4368)
  line L552 (147.0446, 166.1129) -> (147.2594, 166.7408)
  line L553 (146.9906, 171.4887) -> (148.9626, 172.6273)
  line L554 (135.9143, 169.6272) -> (135.8122, 169.1075)
  line L555 (132.8789, 171.3797) -> (132.9342, 171.4483)
  line L556 (136.0801, 169.9314) -> (135.9461, 169.7094)
  line L557 (124.4174, 187.6547) -> (124.2703, 186.8208)
  line L558 (133.0595, 171.6754) -> (133.722, 172.4252)
  line L559 (135.7933, 168.1365) -> (136.0114, 166.7408)
  line L560 (124.7067, 186.3209) -> (125.8064, 185.4341)
  line L561 (124.2703, 179.2617) -> (124.4174, 178.4278)
  line L562 (139.8829, 168.5638) -> (139.8965, 168.6509)
  line L563 (124.4174, 178.4278) -> (124.707, 177.6321)
  line L564 (130.3307, 170.0205) -> (131.6485, 170.5295)
  line L565 (128.6146, 171.7367) -> (128.4866, 171.0855)
  line L566 (139.8965, 168.6509) -> (139.8914, 168.9102)
  line L567 (125.8064, 185.4341) -> (126.6568, 184.9651)
  line L568 (126.6568, 181.1174) -> (125.8064, 180.6484)
  line L569 (139.7115, 168.0627) -> (139.8829, 168.5638)
  line L570 (133.722, 172.4252) -> (134.3081, 172.6273)
  line L571 (150.7908, 171.0314) -> (151.6222, 170.5295)
  line L572 (143.3879, 168.5638) -> (143.5593, 168.0627)
  line L573 (132.9342, 171.4483) -> (133.0595, 171.6754)
  line L574 (129.6255, 173.8858) -> (129.1236, 173.0544)
  line L575 (131.6485, 170.5295) -> (132.4799, 171.0314)
  line L576 (129.6796, 169.8926) -> (130.3307, 170.0205)
  line L577 (139.2424, 167.2123) -> (139.7115, 168.0627)
  line L578 (139.8914, 168.9102) -> (140.0902, 169.8908)
  line L579 (132.4799, 171.0314) -> (132.8789, 171.3797)
  line L580 (49.8277, 176.7057) -> (48.9192, 176.1183)
  line L581 (53.4245, 165.636) -> (54.3231, 165.7482)
  line L582 (50.9257, 180.843) -> (51.4723, 180.7576)
  line L583 (56.265, 162.3847) -> (55.7185, 161.6626)
  line L584 (57.8297, 164.0148) -> (57.5753, 163.7044)
  line L585 (52.7131, 177.9958) -> (52.3544, 177.8157)
  line L586 (51.216, 168.1111) -> (50.5852, 167.3885)
  line L587 (53.7152, 170.2053) -> (53.2507, 169.905)
  line L588 (52.6346, 180.4522) -> (52.8726, 178.1876)
  line L589 (57.8023, 158.7946) -> (58.6579, 159.0911)
  line L590 (56.1211, 166.2232) -> (56.5171, 166.2882)
  line L591 (50.6207, 177.1431) -> (49.8277, 176.7057)
  line L592 (52.8726, 178.1876) -> (52.7131, 177.9958)
  line L593 (56.7589, 166.2269) -> (57.8975, 164.2549)
  line L594 (47.4156, 183.0412) -> (47.4672, 182.0578)
  line L595 (55.197, 159.0927) -> (55.8167, 158.3274)
  line L596 (57.5753, 163.7044) -> (57.1366, 163.3246)
  line L597 (57.1366, 163.3246) -> (56.7447, 162.9343)
  line L598 (53.2507, 169.905) -> (52.6672, 169.4672)
  line L599 (52.6672, 169.4672) -> (51.9825, 168.8745)
  line L600 (57.8975, 164.2549) -> (57.8297, 164.0148)
  line L601 (55.5729, 166.0331) -> (56.1211, 166.2232)
  line L602 (54.2233, 170.4856) -> (53.7152, 170.2053)
  line L603 (55.7185, 161.6626) -> (55.1274, 160.7565)
  line L604 (54.6528, 170.9571) -> (54.5366, 170.7364)
  line L605 (50.5852, 167.3885) -> (50.9381, 166.4692)
  line L606 (55.1274, 160.7565) -> (54.6607, 159.9186)
  line L607 (52.3442, 165.5771) -> (53.4245, 165.636)
  line L608 (58.6579, 159.0911) -> (59.3288, 159.3775)
  line L609 (51.3852, 165.5918) -> (52.3442, 165.5771)
  line L610 (51.2824, 177.45) -> (50.6207, 177.1431)
  line L611 (56.5171, 166.2882) -> (56.7589, 166.2269)
  line L612 (56.7447, 162.9343) -> (56.265, 162.3847)
  line L613 (51.9825, 168.8745) -> (51.216, 168.1111)
  line L614 (54.6607, 159.9186) -> (55.197, 159.0927)
  line L615 (53.9492, 173.1228) -> (54.6528, 170.9571)
  line L616 (50.5647, 173.238) -> (51.4671, 173.161)
  line L617 (54.5366, 170.7364) -> (54.2233, 170.4856)
  line L618 (52.3544, 177.8157) -> (51.7992, 177.6472)
  line L619 (48.306, 174.5701) -> (48.5608, 173.6189)
  line L620 (59.3288, 159.3775) -> (59.8211, 159.6297)
  line L621 (50.9381, 166.4692) -> (51.3852, 165.5918)
  line L622 (56.7579, 158.5124) -> (57.8023, 158.7946)
  line L623 (64.8787, 153.9006) -> (65.3079, 154.2496)
  line L624 (55.0388, 165.8889) -> (55.5729, 166.0331)
  line L625 (55.8167, 158.3274) -> (56.7579, 158.5124)
  line L626 (68.1906, 153.3237) -> (68.0845, 152.9366)
  line L627 (64.2821, 153.481) -> (64.8787, 153.9006)
  line L628 (62.264, 157.7683) -> (61.9139, 157.3056)
  line L629 (61.9139, 157.3056) -> (61.6116, 156.8423)
  line L630 (54.3231, 165.7482) -> (55.0388, 165.8889)
  line L631 (61.6617, 152.1432) -> (62.5439, 152.5198)
  line L632 (62.4647, 158.3737) -> (62.4483, 158.1248)
  line L633 (60.2002, 153.4592) -> (60.8965, 152.7629)
  line L634 (61.2567, 156.2051) -> (60.8723, 155.3851)
  line L635 (60.6917, 160.0756) -> (60.941, 160.066)
  line L636 (59.8211, 159.6297) -> (60.3178, 159.9295)
  line L637 (60.8723, 155.3851) -> (60.4825, 154.3759)
  line L638 (61.6116, 156.8423) -> (61.2567, 156.2051)
  line L639 (67.4242, 151.1982) -> (67.2186, 150.3162)
  line L640 (66.0668, 154.8667) -> (66.3126, 154.909)
  line L641 (67.0472, 149.248) -> (66.9616, 148.2926)
  line L642 (66.3126, 154.909) -> (68.1548, 153.5706)
  line L643 (68.1548, 153.5706) -> (68.1906, 153.3237)
  line L644 (69.4494, 147.861) -> (70.2888, 148.5436)
  line L645 (72.6391, 150.9816) -> (74.7193, 150.0554)
  line L646 (74.8056, 149.8214) -> (74.7823, 149.4207)
  line L647 (66.9616, 148.2926) -> (67.7875, 147.7563)
  line L648 (65.3079, 154.2496) -> (65.7314, 154.6462)
  line L649 (63.5068, 153.013) -> (64.2821, 153.481)
  line L650 (62.5439, 152.5198) -> (63.5068, 153.013)
  line L651 (60.941, 160.066) -> (62.4647, 158.3737)
  line L652 (74.7823, 149.4207) -> (74.6506, 148.8556)
  line L653 (67.2186, 150.3162) -> (67.0472, 149.248)
  line L654 (68.0845, 152.9366) -> (67.8382, 152.4113)
  line L655 (60.4825, 154.3759) -> (60.2002, 153.4592)
  line L656 (71.7934, 150.1277) -> (72.1252, 150.6037)
  line L657 (60.3178, 159.9295) -> (60.6917, 160.0756)
  line L658 (60.8965, 152.7629) -> (61.6617, 152.1432)
  line L659 (74.7193, 150.0554) -> (74.8056, 149.8214)
  line L660 (62.4483, 158.1248) -> (62.264, 157.7683)
  line L661 (70.9498, 149.1626) -> (71.4462, 149.6971)
  line L662 (72.4074, 150.8891) -> (72.6391, 150.9816)
  line L663 (67.6389, 151.8952) -> (67.4242, 151.1982)
  line L664 (65.7314, 154.6462) -> (66.0668, 154.8667)
  line L665 (67.8382, 152.4113) -> (67.6389, 151.8952)
  line L666 (72.1252, 150.6037) -> (72.4074, 150.8891)
  line L667 (67.7875, 147.7563) -> (68.6649, 147.3093)
  line L668 (68.6649, 147.3093) -> (69.4494, 147.861)
  line L669 (71.4462, 149.6971) -> (71.7934, 150.1277)
  line L670 (70.2888, 148.5436) -> (70.9498, 149.1626)
  line L671 (79.6438, 217.6272) -> (79.4364, 217.7658)
  line L672 (74.6495, 221.4378) -> (74.5346, 220.4855)
  line L673 (86.705, 219.1961) -> (86.5955, 219.7659)
  line L674 (81.8712, 218.1006) -> (79.6438, 217.6272)
  line L675 (93.3908, 223.4076) -> (92.4182, 223.5616)
  line L676 (89.4719, 218.8206) -> (89.2978, 218.6419)
  line L677 (75.5688, 221.7907) -> (74.6495, 221.4378)
  line L678 (71.4462, 216.3855) -> (70.9498, 216.9199)
  line L679 (82.1686, 220.5651) -> (82.0812, 219.841)
  line L680 (82.0812, 219.841) -> (82.0534, 219.2885)
  line L681 (86.8467, 218.8206) -> (86.705, 219.1961)
  line L682 (72.6391, 215.1009) -> (72.4074, 215.1934)
  line L683 (74.6506, 217.2269) -> (74.7823, 216.6619)
  line L684 (72.1252, 215.4789) -> (71.7934, 215.9548)
  line L685 (86.5955, 219.7659) -> (86.4534, 220.3005)
  line L686 (94.3144, 218.3116) -> (94.2539, 218.7084)
  line L687 (74.8056, 216.2612) -> (74.7193, 216.0271)
  line L688 (83.9004, 223.5616) -> (82.9278, 223.4076)
  line L689 (86.2174, 220.9907) -> (85.8653, 221.825)
  line L690 (89.2978, 218.6419) -> (87.0207, 218.6419)
  line L691 (78.9942, 218.6383) -> (78.7441, 219.1317)
  line L692 (74.5346, 220.4855) -> (74.4802, 219.4051)
  line L693 (71.7934, 215.9548) -> (71.4462, 216.3855)
  line L694 (70.2888, 217.5389) -> (69.4494, 218.2215)
  line L695 (89.6135, 219.1961) -> (89.4719, 218.8206)
  line L696 (79.2198, 218.1037) -> (78.9942, 218.6383)
  line L697 (74.4802, 219.4051) -> (74.4978, 218.4996)
  line L698 (67.0472, 216.8345) -> (67.2186, 215.7664)
  line L699 (77.1727, 221.3427) -> (76.52, 222.0456)
  line L700 (72.4074, 215.1934) -> (72.1252, 215.4789)
  line L701 (74.7193, 216.0271) -> (72.6391, 215.1009)
  line L702 (70.9498, 216.9199) -> (70.2888, 217.5389)
  line L703 (82.0647, 218.7084) -> (82.0042, 218.3116)
  line L704 (79.4364, 217.7658) -> (79.2198, 218.1037)
  line L705 (82.9278, 223.4076) -> (82.6174, 222.5)
  line L706 (76.52, 222.0456) -> (75.5688, 221.7907)
  line L707 (74.7823, 216.6619) -> (74.8056, 216.2612)
  line L708 (86.4534, 220.3005) -> (86.2174, 220.9907)
  line L709 (89.8651, 220.3005) -> (89.7231, 219.7659)
  line L710 (91.4348, 223.6132) -> (90.9425, 222.79)
  line L711 (94.2652, 219.2885) -> (94.2374, 219.841)
  line L712 (74.4978, 218.4996) -> (74.5629, 217.7731)
  line L713 (78.7441, 219.1317) -> (78.3697, 219.7577)
  line L714 (82.0042, 218.3116) -> (81.8712, 218.1006)
  line L715 (74.5629, 217.7731) -> (74.6506, 217.2269)
  line L716 (82.6174, 222.5) -> (82.3396, 221.4545)
  line L717 (84.8838, 223.6132) -> (83.9004, 223.5616)
  line L718 (77.8518, 220.5006) -> (77.1727, 221.3427)
  line L719 (82.0534, 219.2885) -> (82.0647, 218.7084)
  line L720 (78.3697, 219.7577) -> (77.8518, 220.5006)
  line L721 (68.0845, 213.1459) -> (68.1906, 212.7588)
  line L722 (67.7875, 218.3262) -> (66.9616, 217.7899)
  line L723 (65.7314, 211.4364) -> (65.3079, 211.8329)
  line L724 (67.4242, 214.8844) -> (67.6389, 214.1873)
  line L725 (63.5068, 213.0696) -> (62.5439, 213.5627)
  line L726 (67.2186, 215.7664) -> (67.4242, 214.8844)
  line L727 (60.4825, 211.7066) -> (60.8723, 210.6974)
  line L728 (67.8382, 213.6713) -> (68.0845, 213.1459)
  line L729 (61.6617, 213.9393) -> (60.8965, 213.3196)
  line L730 (69.4494, 218.2215) -> (68.6649, 218.7733)
  line L731 (61.6116, 209.2402) -> (61.9139, 208.7769)
  line L732 (67.6389, 214.1873) -> (67.8382, 213.6713)
  line L733 (60.2002, 212.6233) -> (60.4825, 211.7066)
  line L734 (66.0668, 211.2158) -> (65.7314, 211.4364)
  line L735 (68.1906, 212.7588) -> (68.1548, 212.512)
  line L736 (61.9139, 208.7769) -> (62.264, 208.3143)
  line L737 (68.6649, 218.7733) -> (67.7875, 218.3262)
  line L738 (62.264, 208.3143) -> (62.4483, 207.9577)
  line L739 (62.5439, 213.5627) -> (61.6617, 213.9393)
  line L740 (66.3126, 211.1735) -> (66.0668, 211.2158)
  line L741 (61.2567, 209.8775) -> (61.6116, 209.2402)
  line L742 (64.2821, 212.6016) -> (63.5068, 213.0696)
  line L743 (60.941, 206.0166) -> (60.6917, 206.0068)
  line L744 (66.9616, 217.7899) -> (67.0472, 216.8345)
  line L745 (62.4483, 207.9577) -> (62.4647, 207.7088)
  line L746 (64.8787, 212.182) -> (64.2821, 212.6016)
  line L747 (68.1548, 212.512) -> (66.3126, 211.1735)
  line L748 (60.8723, 210.6974) -> (61.2567, 209.8775)
  line L749 (65.3079, 211.8329) -> (64.8787, 212.182)
  line L750 (62.4647, 207.7088) -> (60.941, 206.0166)
  line L751 (60.8965, 213.3196) -> (60.2002, 212.6233)
  line L752 (57.8297, 202.0676) -> (57.8975, 201.8275)
  line L753 (54.3231, 200.3342) -> (53.4245, 200.4464)
  line L754 (57.5753, 202.3781) -> (57.8297, 202.0676)
  line L755 (54.6607, 206.1638) -> (55.1274, 205.3259)
  line L756 (57.8975, 201.8275) -> (56.7589, 199.8555)
  line L757 (56.1211, 199.8592) -> (55.5729, 200.0493)
  line L758 (58.6579, 206.9912) -> (57.8023, 207.2878)
  line L759 (55.7185, 204.4198) -> (56.265, 203.6977)
  line L760 (56.7579, 207.57) -> (55.8167, 207.755)
  line L761 (56.265, 203.6977) -> (56.7447, 203.1482)
  line L762 (56.5171, 199.7942) -> (56.1211, 199.8592)
  line L763 (55.5729, 200.0493) -> (55.0388, 200.1935)
  line L764 (55.1274, 205.3259) -> (55.7185, 204.4198)
  line L765 (59.8211, 206.4527) -> (59.3288, 206.7049)
  line L766 (50.9381, 199.6131) -> (50.5852, 198.6938)
  line L767 (55.0388, 200.1935) -> (54.3231, 200.3342)
  line L768 (53.4245, 200.4464) -> (52.3442, 200.5053)
  line L769 (51.3852, 200.4905) -> (50.9381, 199.6131)
  line L770 (51.216, 197.9712) -> (51.9825, 197.2078)
  line L771 (52.3442, 200.5053) -> (51.3852, 200.4905)
  line L772 (51.9825, 197.2078) -> (52.6672, 196.6151)
  line L773 (52.6672, 196.6151) -> (53.2507, 196.1773)
  line L774 (55.8167, 207.755) -> (55.197, 206.9897)
  line L775 (56.7589, 199.8555) -> (56.5171, 199.7942)
  line L776 (59.3288, 206.7049) -> (58.6579, 206.9912)
  line L777 (60.3178, 206.1528) -> (59.8211, 206.4527)
  line L778 (56.7447, 203.1482) -> (57.1366, 202.7578)
  line L779 (50.5852, 198.6938) -> (51.216, 197.9712)
  line L780 (60.6917, 206.0068) -> (60.3178, 206.1528)
  line L781 (55.197, 206.9897) -> (54.6607, 206.1638)
  line L782 (53.3245, 192.8307) -> (52.7488, 192.9026)
  line L783 (50.5647, 192.8443) -> (49.4959, 192.6773)
  line L784 (51.4723, 185.3247) -> (50.9257, 185.2393)
  line L785 (54.6528, 195.1252) -> (53.9492, 192.9596)
  line L786 (54.5366, 195.346) -> (54.6528, 195.1252)
  line L787 (53.2507, 196.1773) -> (53.7152, 195.877)
  line L788 (48.306, 191.5122) -> (48.1519, 190.5397)
  line L789 (52.6346, 185.6301) -> (52.4387, 185.4758)
  line L790 (52.0504, 185.3741) -> (51.4723, 185.3247)
  line L791 (54.2233, 195.5967) -> (54.5366, 195.346)
  line L792 (53.7152, 195.877) -> (54.2233, 195.5967)
  line L793 (53.9492, 192.9596) -> (53.7254, 192.8493)
  line L794 (57.1366, 202.7578) -> (57.5753, 202.3781)
  line L795 (51.2824, 188.6323) -> (51.7992, 188.4352)
  line L796 (57.8023, 207.2878) -> (56.7579, 207.57)
  line L797 (52.3544, 188.2667) -> (52.7131, 188.0865)
  line L798 (52.4387, 180.6066) -> (52.6346, 180.4522)
  line L799 (51.7992, 188.4352) -> (52.3544, 188.2667)
  line L800 (50.6207, 188.9392) -> (51.2824, 188.6323)
  line L801 (52.1964, 173.1497) -> (52.7488, 173.1798)
  line L802 (47.4672, 182.0578) -> (48.3373, 181.6542)
  line L803 (49.3481, 181.2686) -> (50.2147, 181.0056)
  line L804 (48.3373, 184.4281) -> (47.4672, 184.0246)
  line L805 (50.9257, 185.2393) -> (50.2147, 185.0767)
  line L806 (52.7131, 188.0865) -> (52.8726, 187.8948)
  line L807 (52.4387, 185.4758) -> (52.0504, 185.3741)
  line L808 (50.2147, 185.0767) -> (49.3481, 184.8137)
  line L809 (49.4959, 173.4051) -> (50.5647, 173.238)
  line L810 (49.3481, 184.8137) -> (48.3373, 184.4281)
  line L811 (48.1519, 190.5397) -> (48.9192, 189.964)
  line L812 (53.7254, 192.8493) -> (53.3245, 192.8307)
  line L813 (52.1964, 192.9327) -> (51.4671, 192.9214)
  line L814 (49.4959, 192.6773) -> (48.5608, 192.4634)
  line L815 (49.8277, 189.3766) -> (50.6207, 188.9392)
  line L816 (52.7488, 192.9026) -> (52.1964, 192.9327)
  line L817 (48.5608, 192.4634) -> (48.306, 191.5122)
  line L818 (48.9192, 189.964) -> (49.8277, 189.3766)
  line L819 (52.8726, 187.8948) -> (52.6346, 185.6301)
  line L820 (51.4671, 192.9214) -> (50.5647, 192.8443)
  line L821 (48.1519, 175.5427) -> (48.306, 174.5701)
  line L822 (48.3373, 181.6542) -> (49.3481, 181.2686)
  line L823 (48.5608, 173.6189) -> (49.4959, 173.4051)
  line L824 (53.7254, 173.233) -> (53.9492, 173.1228)
  line L825 (50.2147, 181.0056) -> (50.9257, 180.843)
  line L826 (51.7992, 177.6472) -> (51.2824, 177.45)
  line L827 (51.4671, 173.161) -> (52.1964, 173.1497)
  line L828 (52.0504, 180.7082) -> (52.4387, 180.6066)
  line L829 (51.4723, 180.7576) -> (52.0504, 180.7082)
  line L830 (48.9192, 176.1183) -> (48.1519, 175.5427)
  line L831 (52.7488, 173.1798) -> (53.3245, 173.2516)
  line L832 (53.3245, 173.2516) -> (53.7254, 173.233)
  line L833 (47.4672, 184.0246) -> (47.4156, 183.0412)